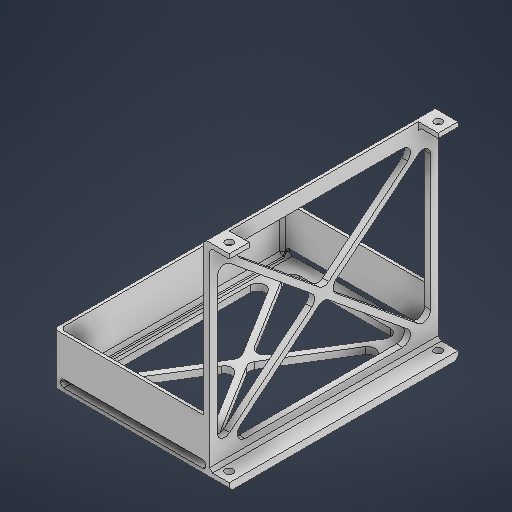
# Autodesk Inventor part: HolderWater
Saved by Autodesk Inventor 2025.1 (Build 291241000, 241)
## iProperties
Created: 2025-11-23
Part Number: HolderWater
Material: Типовые
Document SubType Name: Modeling
Designer: bogda
Density: 1 g/cm^3
Appearance: По умолчанию
Author: bogda
Autodesk Inventor part; units mm, degrees
ref_plane "YZ Plane" through (0, 0, 0) normal (1, 0, 0) x (0, 1, 0)
ref_plane "XZ Plane" through (0, 0, 0) normal (0, 1, 0) x (-1, 0, 0)
ref_plane "XY Plane" through (0, 0, 0) normal (0, 0, 1) x (1, 0, 0)
sketch "Эскиз1" plane through (0, 0, 0) normal (0, 1, 0) x (-1, 0, 0)
  line L0 (0, 0) -> (100, 0)
  line L1 (100, 0) -> (100, -150)
  line L2 (100, -150) -> (0, -150)
  line L3 (98, -148) -> (98, -2)
  line L4 (98, -2) -> (2, -2)
  line L5 (2, -2) -> (2, -148)
  line L6 (2, -148) -> (98, -148)
  line L7 (0, 0) -> (-15, 0)
  line L8 (-15, 0) -> (-15, -150)
  line L9 (-15, -150) -> (0, -150)
  line L10 (2, 0) -> (-2, 0)
  line L11 (-2, 0) -> (-2, -150)
  line L12 (-2, -150) -> (2, -150)
  line L13 (2, -150) -> (2, 0)
  dimension "d0" = 100
  dimension "d1" = 150
  dimension "d2" = 2
  dimension "d3" = 15
  dimension "d4" = 4
  constraints: 28 end point, 6 parallel, 4 perpendicular, 3 horizontal, 2 point on line, 1 other
  measures "d0" distance of L1.end L2.end
  measures "d1" distance of L0.end L1.end
  measures "d2" distance between parallel lines of L1 L3
  measures "d3" distance of L9.end L8.end
  measures "d4" distance of L12.end L11.end
extrude "Выдавливание1" add sketch "Эскиз1" along normal blind 30 contours L0 L1 L2 L13 L6 L3 L4
extrude "Выдавливание2" add sketch "Эскиз1" along normal blind 130 contours L0 L13 L5 L2 L9 L11 L7
extrude "Выдавливание3" add sketch "Эскиз1" against normal blind 5
sketch "Эскиз2" plane through (0, 130, 0) normal (0, 1, 0) x (1, 0, 0)
  line L0 (2, 0) -> (2, 150) projected
  line L1 (15, 0) -> (15, 150) projected
  line L2 (2, 0) -> (15, 0)
  line L3 (15, 0) -> (15, 13)
  line L4 (15, 13) -> (2, 13)
  line L5 (2, 13) -> (2, 0)
  line L6 (15, 0) -> (2, 13)
  line L7 (15, 13) -> (2, 0)
  circle A0 centre (8.5, 6.5) radius 2.6
  line L8 (15, 150) -> (2, 150) projected
  line L9 (2, 150) -> (15, 150)
  line L10 (15, 150) -> (15, 137)
  line L11 (15, 137) -> (2, 137)
  line L12 (2, 137) -> (2, 150)
  line L13 (15, 137) -> (2, 150)
  line L14 (2, 150) -> (-2, 150) projected
  line L15 (2, 137) -> (15, 150)
  circle A1 centre (8.5, 143.5) radius 2.6
  point P0 (0, 0)
  point P1 (2, 13)
  dimension "d11" = 13
  dimension "d12" = 5.2
  dimension "d13" = 13
  dimension "d14" = 5.2
  constraints: 24 end point, 4 parallel, 3 perpendicular, 3 point on line, 2 centre point, 2 horizontal, 2 midpoint
  measures "d11" distance of L3.end L2.end
  measures "d12" diameter of A0
  measures "d13" distance of L9.end L10.end
  measures "d14" diameter of A1
extrude "Выдавливание4" add sketch "Эскиз2" against normal blind 3 contours L7 A0 L6 L2 | L0 L6 A0 L7 | L4 L7 A0 L6 | L6 A0 L7 L1 | L15 A1 L13 L11 | L0 L13 A1 L15 | L8 L15 A1 L13 | L13 A1 L15 L1
extrude "Выдавливание5" cut sketch "Эскиз2" against normal blind 150 contours A0 L6 L7 | L7 L6 A0 | A0 L7 L6 | L6 L7 A0 | A1 L13 L15 | L15 L13 A1 | A1 L15 L13 | L13 L15 A1
chamfer "Фаска1" distance 2 angle 45 17 edges at (-100, 12.5, -150) (-98, 15, -2) (-98, 0, -75) (-50, 0, -2) (-100, 12.5, 0) (-50, 0, -148) (-98, 15, -148) (-2, 0, -75) (-2, 15, -148) (-2, 15, -2) (-42.5, -5, -150) (-100, -5, -75) (-42.5, -5, 0) (2, 0, -75) (-2, 130, -75) (2, 127, -6.5) (2, 127, -143.5)
sketch "Эскиз3" plane through (2, 130, -13) normal (1, 0, 0) x (0, 0, -1)
  line L0 (-13, -5) -> (0, -5) projected
  line L1 (137, -128) -> (-13, -128) projected
  line L2 (-13, -5) -> (137, -5)
  line L3 (137, -5) -> (137, -128)
  line L4 (137, -128) -> (-13, -128)
  line L5 (-13, -128) -> (-13, -5)
  line L6 (113.7653, -123) -> (10.2347, -123)
  line L7 (10.2347, -10) -> (113.7653, -10)
  line L8 (132, -22.2525) -> (132, -110.7475)
  line L9 (-9.8458, -128) -> (-11.7318, -129.5465)
  line L10 (-8, -110.7475) -> (-8, -22.2525)
  line L11 (7.0643, -18.8663) -> (58.8296, -61.3138)
  line L12 (69.8692, -70.3663) -> (123.8296, -114.6138)
  line L13 (116.9357, -18.8663) -> (65.1704, -61.3138)
  line L14 (54.1308, -70.3663) -> (0.1704, -114.6138)
  line L15 (123.8296, -18.3862) -> (69.8692, -62.6337)
  line L16 (58.8296, -71.6862) -> (7.0643, -114.1337)
  line L17 (0.1704, -18.3862) -> (54.1308, -62.6337)
  line L18 (65.1704, -71.6862) -> (116.9357, -114.1337)
  arc A0 (60.7318, -62.8737) -> (63.2682, -62.8737) centre (62, -61.3271) ccw
  arc A1 (69.8692, -62.6337) -> (69.8692, -70.3663) centre (73.0396, -66.5) ccw
  arc A2 (58.8296, -61.3138) -> (65.1704, -61.3138) centre (62, -57.4475) ccw
  arc A3 (54.1308, -70.3663) -> (54.1308, -62.6337) centre (50.9604, -66.5) ccw
  arc A4 (65.1704, -71.6862) -> (58.8296, -71.6862) centre (62, -75.5525) ccw
  arc A5 (123.8296, -114.6138) -> (132, -110.7475) centre (127, -110.7475) ccw
  arc A6 (113.7653, -123) -> (116.9357, -114.1337) centre (113.7653, -118) ccw
  arc A7 (7.0643, -114.1337) -> (10.2347, -123) centre (10.2347, -118) ccw
  arc A8 (-8, -110.7475) -> (0.1704, -114.6138) centre (-3, -110.7475) ccw
  arc A9 (0.1704, -18.3862) -> (-8, -22.2525) centre (-3, -22.2525) ccw
  arc A10 (10.2347, -10) -> (7.0643, -18.8663) centre (10.2347, -15) ccw
  arc A11 (116.9357, -18.8663) -> (113.7653, -10) centre (113.7653, -15) ccw
  arc A12 (132, -22.2525) -> (123.8296, -18.3862) centre (127, -22.2525) ccw
  point P0 (-13, -130)
  dimension "d29" = 5
  dimension "d30" = 2
  dimension "d31" = 5
  constraints: 34 end point, 26 point on circle, 26 tangent, 13 centre point, 11 equal radius, 6 parallel, 3 point on line, 1 horizontal, 1 perpendicular
  measures "d29" distance between parallel lines of L1 L6
  measures "d30" radius of A0
  measures "d31" radius of A1
extrude "Выдавливание6" cut sketch "Эскиз3" against normal blind 50 contours L6 A7 L16 A4 L18 A6 | L7 A11 L13 A2 L11 A10 | L8 A5 L12 A1 L15 A12 | L10 A9 L17 A3 L14 A8
sketch "Эскиз4" plane through (0, 0, 0) normal (0, 1, 0) x (1, 0, 0)
  line L0 (-4, 146) -> (-4, 148) projected
  line L1 (-4, 146) -> (-96, 146)
  line L2 (-96, 146) -> (-96, 4)
  line L3 (-96, 4) -> (-4, 4)
  line L4 (-4, 4) -> (-4, 146)
  line L5 (-20.3468, 141) -> (-79.6532, 141)
  line L6 (-91, 119.6857) -> (-91, 30.3143)
  line L7 (-79.6532, 9) -> (-20.3468, 9)
  line L8 (-9, 30.3143) -> (-9, 119.6857)
  line L9 (-18.2472, 27.6759) -> (-46.0065, 72.3616)
  line L10 (-54.2472, 85.6271) -> (-83.9004, 133.3616)
  line L11 (-16.0996, 16.6384) -> (-45.7528, 64.3729)
  line L12 (-53.9935, 77.6384) -> (-81.7528, 122.3241)
  line L13 (-16.0996, 133.3616) -> (-45.7528, 85.6271)
  line L14 (-53.9935, 72.3616) -> (-81.7528, 27.6759)
  line L15 (-18.2472, 122.3241) -> (-46.0065, 77.6384)
  line L16 (-54.2472, 64.3729) -> (-83.9004, 16.6384)
  arc A0 (-46.0065, 77.6384) -> (-46.0065, 72.3616) centre (-41.7593, 75) ccw
  arc A1 (-45.7528, 64.3729) -> (-54.2472, 64.3729) centre (-50, 61.7345) ccw
  arc A2 (-53.9935, 72.3616) -> (-53.9935, 77.6384) centre (-58.2407, 75) ccw
  arc A3 (-54.2472, 85.6271) -> (-45.7528, 85.6271) centre (-50, 88.2655) ccw
  arc A4 (-9, 119.6857) -> (-18.2472, 122.3241) centre (-14, 119.6857) ccw
  arc A5 (-18.2472, 27.6759) -> (-9, 30.3143) centre (-14, 30.3143) ccw
  arc A6 (-20.3468, 9) -> (-16.0996, 16.6384) centre (-20.3468, 14) ccw
  arc A7 (-83.9004, 16.6384) -> (-79.6532, 9) centre (-79.6532, 14) ccw
  arc A8 (-91, 30.3143) -> (-81.7528, 27.6759) centre (-86, 30.3143) ccw
  arc A9 (-81.7528, 122.3241) -> (-91, 119.6857) centre (-86, 119.6857) ccw
  arc A10 (-79.6532, 141) -> (-83.9004, 133.3616) centre (-79.6532, 136) ccw
  arc A11 (-16.0996, 133.3616) -> (-20.3468, 141) centre (-20.3468, 136) ccw
  point P0 (0, 0)
  dimension "d34" = 5
  dimension "d39" = 5
  constraints: 32 end point, 24 point on circle, 24 tangent, 12 centre point, 11 equal radius, 4 parallel, 2 perpendicular, 1 horizontal
  measures "d34" distance between parallel lines of L4 L8
  measures "d39" radius of A0
extrude "Выдавливание7" cut sketch "Эскиз4" against normal blind 50 contours A11 L13 A3 L10 A10 L5 | A9 L12 A2 L14 A8 L6 | A7 L16 A1 L11 A6 L7 | A5 L9 A0 L15 A4 L8
sketch "Эскиз5" plane through (4, 0, 0) normal (0, 0, 1) x (1, 0, 0)
  line L0 (-102, 30) -> (-102, -3) projected
  line L1 (-2, 2) -> (-2, 125) projected
  line L2 (-102, -3) -> (-2, -3)
  line L3 (-2, -3) -> (-2, 7)
  line L4 (-2, 7) -> (-102, 7)
  line L5 (-102, 7) -> (-102, -3)
  line L6 (-97.5, 4.5) -> (-6.5, 4.5)
  line L7 (-4.5, 2.5) -> (-4.5, 1.5)
  line L8 (-6.5, -0.5) -> (-97.5, -0.5)
  line L9 (-99.5, 1.5) -> (-99.5, 2.5)
  arc A0 (-97.5, 4.5) -> (-99.5, 2.5) centre (-97.5, 2.5) ccw
  arc A1 (-99.5, 1.5) -> (-97.5, -0.5) centre (-97.5, 1.5) ccw
  arc A2 (-4.5, 2.5) -> (-6.5, 4.5) centre (-6.5, 2.5) ccw
  arc A3 (-6.5, -0.5) -> (-4.5, 1.5) centre (-6.5, 1.5) ccw
  point P0 (-4, 0)
  dimension "d42" = 10
  dimension "d43" = 2.5
  dimension "d44" = 2
  constraints: 16 end point, 8 point on circle, 8 tangent, 4 centre point, 4 parallel, 3 equal radius, 2 perpendicular, 1 horizontal, 1 point on line, 3 other
  measures "d42" distance of L3.end L2.end
  measures "d43" distance between parallel lines of L4 L6
  measures "d44" radius of A0
extrude "Выдавливание8" cut sketch "Эскиз5" against normal blind 1111 contours L6 A2 L7 A3 L8 A1 L9 A0
